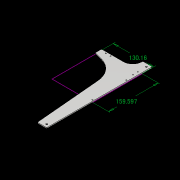
# Autodesk Inventor part: small_gpu_05
Saved by Autodesk Inventor 2018.2 (Build 222227000, 227)
## iProperties
Created: 2020-06-13
Part Number: small_gpu_05
Material: アルミニウム 6061
Document SubType Name: Modeling
Designer: gisen
Density: 2.7 g/cm^3
Appearance: アルミニウム - フラット
Author: gisen
Autodesk Inventor part; units mm, degrees
ref_plane "YZ Plane" through (0, 0, 0) normal (1, 0, 0) x (0, 1, 0)
ref_plane "XZ Plane" through (0, 0, 0) normal (0, 1, 0) x (-1, 0, 0)
ref_plane "XY Plane" through (0, 0, 0) normal (0, 0, 1) x (1, 0, 0)
sketch "スケッチ1" plane through (0, 0, 0) normal (0, 0, 1) x (1, 0, 0)
  line L0 (0, 0) -> (130.16, 0)
  line L1 (130.16, 0) -> (130.16, 159.597)
  line L2 (130.16, 159.597) -> (0, 159.597)
  line L3 (0, 159.597) -> (0, 0)
  dimension "d0" = 130.16
  dimension "d1" = 159.597
  constraints: 8 end point, 2 parallel, 1 horizontal, 1 perpendicular
  measures "d0" distance of L1.end L2.end
  measures "d1" distance between parallel lines of L0 L2
extrude "押し出し1" add sketch "スケッチ1" along normal blind 3
sketch "スケッチ2" plane through (0, 0, 3) normal (0, 0, 1) x (1, 0, 0)
  line L0 (126.16, 3.92) -> (126.16, 113.08) construction
  circle A0 centre (126.16, 3.92) radius 1.6
  circle A1 centre (126.16, 113.08) radius 1.6
  line L1 (130.16, 0) -> (130.16, 159.597) projected
  line L2 (0, 0) -> (130.16, 0) projected
  circle A2 centre (121.531, 154.597) radius 1.6
  line L3 (130.16, 159.597) -> (0, 159.597) projected
  line L4 (121.531, 154.597) -> (121.531, 139.097) construction
  circle A3 centre (121.531, 139.097) radius 1.6
  line L5 (18.398, 154.597) -> (33.898, 154.597) construction
  line L6 (0, 159.597) -> (0, 0) construction
  circle A4 centre (18.398, 154.597) radius 1.6
  circle A5 centre (33.898, 154.597) radius 1.6
  dimension "d4" = 3.2
  dimension "d5" = 4
  dimension "d6" = 3.92
  dimension "d7" = 109.16
  dimension "d10" = 5
  dimension "d11" = 8.629
  dimension "d12" = 15.5
  dimension "d13" = 18.398
  dimension "d14" = 5
  dimension "d15" = 15.5
  constraints: 6 centre point, 6 end point, 5 coincident, 5 equal radius, 2 vertical, 1 horizontal
  measures "d4" diameter of A0
  measures "d5" distance between parallel lines of L1 L0
  measures "d6" distance from line of L2 L0.start
  measures "d7" distance of L0.start L0.end
  measures "d10" distance from line of L4.start L3
  measures "d11" distance from line of L1 L4.start
  measures "d12" distance of L4.start L4.end
  measures "d13" distance from line of L6 L5.start
  measures "d14" distance between parallel lines of L5 L3
  measures "d15" distance of L5.start L5.end
extrude "押し出し2" cut sketch "スケッチ2" against normal blind 3
sketch "スケッチ9" plane through (0, 0, 3) normal (0, 0, 1) x (1, 0, 0)
  line L0 (130.16, 159.597) -> (0, 159.597)
  line L1 (100.16, 192.597) -> (130.16, 192.597)
  line L2 (130.16, 192.597) -> (130.16, 159.597)
  line L3 (100.16, 192.597) -> (100.16, 187.597)
  line L4 (130.16, 159.597) -> (0, 159.597) projected
  line L5 (100.16, 187.597) -> (0, 159.597)
  line L6 (130.16, 0) -> (130.16, -147.403)
  line L7 (130.16, -147.403) -> (100.16, -147.403)
  line L8 (100.16, -147.403) -> (100.16, -142.403)
  line L9 (100.16, -142.403) -> (0, 0)
  line L10 (0, 0) -> (130.16, 0)
  circle A0 centre (120.66, 182.597) radius 2.75
  circle A1 centre (120.66, -137.403) radius 2.75
  line L11 (130.16, 192.097) -> (100.16, 192.097)
  line L12 (130.16, -146.903) -> (100.16, -146.903)
  dimension "d50" = 33
  dimension "d51" = 30
  dimension "d52" = 5
  dimension "d53" = 340
  dimension "d54" = 10
  dimension "d55" = 9.5
  dimension "d56" = 0.5
  dimension "d57" = 5.5
  dimension "d58" = 9.5
  dimension "d59" = 10
  dimension "d60" = 0.5
  constraints: 24 end point, 4 coincident, 4 perpendicular, 4 point on line, 2 centre point, 2 equal length, 2 horizontal, 2 vertical, 1 equal radius, 1 parallel
  measures "d50" distance of L1.end L0.start
  measures "d51" distance of L1.start L1.end
  measures "d52" distance of L1.start L3.end
  measures "d53" distance between parallel lines of L7 L1
  measures "d54" distance from line of A0.centre L1
  measures "d55" distance from line of A0.centre L2
  measures "d56" distance between parallel lines of L1 L11
  measures "d57" diameter of A0
  measures "d58" distance from line of A1.centre L6
  measures "d59" distance from line of L7 A1.centre
  measures "d60" distance between parallel lines of L12 L7
extrude "押し出し8" add sketch "スケッチ9" against normal blind 3 contours L0 L5 L3 L11 L2 | L6 L12 L8 L9 L10
sketch "スケッチ10" plane through (0, 0, 3) normal (0, 0, 1) x (1, 0, 0)
  line L0 (100.16, -146.903) -> (100.16, -142.403) projected
  line L1 (100.16, -142.403) -> (77.3003, 118.8844)
  line L2 (77.3003, 118.8844) -> (0, 139.597)
  line L3 (0, 159.597) -> (0, 0) projected
  line L4 (0, 139.597) -> (0, 0)
  line L5 (0, 0) -> (100.16, -142.403)
  line L6 (130.16, -146.903) -> (130.16, 192.097) projected
  dimension "d63" = 20
  dimension "d64" = 105
  dimension "d65" = 5
  constraints: 9 end point, 1 point on line
  measures "d63" distance of L2.end L3.start
  measures "d64" angle of L3 L2
  measures "d65" angle of L1 L6
extrude "押し出し9" cut sketch "スケッチ10" against normal blind 3
fillet "フィレット2" radius 75 1 edges at (77.3003, 118.8844, 1.5)
sketch "スケッチ12" plane through (0, 0, 3) normal (0, 0, 1) x (1, 0, 0)
  line L0 (100.16, 187.597) -> (100.16, 159.597)
  line L1 (100.16, 159.597) -> (0, 159.597)
  line L2 (0, 159.597) -> (100.16, 187.597)
  line L3 (0, 159.597) -> (0, 139.597) projected
  point P0 (0, 0)
  constraints: 6 end point, 2 coincident, 1 perpendicular
extrude "押し出し10" cut sketch "スケッチ12" against normal blind 3
fillet "フィレット4" radius 30 1 edges at (100.16, 159.597, 1.5)
fillet "フィレット5" radius 2 5 edges at (100.16, 192.097, 1.5) (0, 159.597, 1.5) (100.16, -146.903, 1.5) (130.16, -146.903, 1.5) (130.16, 192.097, 1.5)
equation "\"d58\" = d55"
equation "\"d59\" = d54"
equation "\"d60\" = d56"
